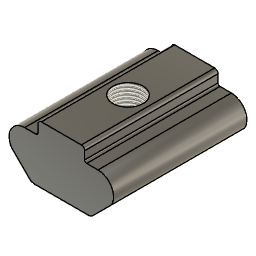
T nut v2 (Autodesk Fusion 360 design; units mm, degrees)
Autodesk Fusion 360 part; units mm, degrees
sketch "Sketch1" plane through (0, 0, 0) normal (0, 1, 0) x (1, 0, 0)
  line L0 (4.45, 0) -> (-4.45, 0)
  line L1 (-3.5, -8.6) -> (3.5, -8.6)
  line L2 (3.5, -8.6) -> (3.5, -6.6)
  line L3 (-3.5, -8.6) -> (-3.5, -6.6)
  line L4 (4.45, 0) -> (7.5, -3.05)
  line L5 (-4.45, 0) -> (-7.5, -3.05)
  line L6 (-4.45, 0) -> (-0.1366, 0) construction
  arc A0 (5.5, -6.6) -> (7.5, -3.05) centre (5.5, -4.2616) ccw
  arc A1 (-7.5, -3.05) -> (-5.5, -6.6) centre (-5.5, -4.2616) ccw
  line L7 (-5.5, -6.6) -> (-3.5, -6.6)
  line L8 (3.5, -6.6) -> (5.5, -6.6)
  dimension "d2" = 8.9
  dimension "d3" = 2
  dimension "d4" = 7
  dimension "d8" = 135
  constraint perpendicular L1 L2
  constraint perpendicular L1 L3
  constraint equal L2 L3
  constraint midpoint origin L0
  constraint horizontal L6
  constraint tangent A1 L7
  constraint tangent A0 L8
  measures "d2" distance of L0.start L0.end
  measures "d3" distance of L1.end L2.end
  measures "d4" distance of L1.start L1.end
  measures "d8" angle of L5 L6
extrude "Extrude3" add sketch "Sketch1" along normal mid plane 20
sketch "Sketch2" plane through (0, 0, 8.6) normal (0, 0, 1) x (-1, 0, 0)
  line L0 (-3.5, 10) -> (-3.5, -10)
  line L1 (-3.5, -10) -> (3.5, -10)
  line L2 (3.5, -10) -> (3.5, 10)
  line L3 (3.5, 10) -> (-3.5, 10)
  circle A0 centre (0, 0) radius 2.5
  dimension "d22" = 5
  constraint coincident A0.centre origin
  measures "d22" diameter of A0
extrude "Extrude4" cut sketch "Sketch2" against normal blind 8.8 contours A0
thread "Thread2" "ISO Metric profile 5.0 M5x0.5 6H" major diameter 5.0861 minor diameter 4.5287 pitch 0.5 angle 60 resizes the face on face at (-2.4876, 0.2489, 5.7333)
fillet "Fillet4" radius 1 2 edges at (4.45, 0, 0) (-4.45, 0, 0)
fillet "Fillet5" radius 0.3 2 edges at (3.5, 0, 6.6) (-3.5, 0, 6.6)
fillet "Fillet6" radius 0.5 2 edges at (-3.5, 0, 8.6) (3.5, 0, 8.6)
named bodies: "Body1"
